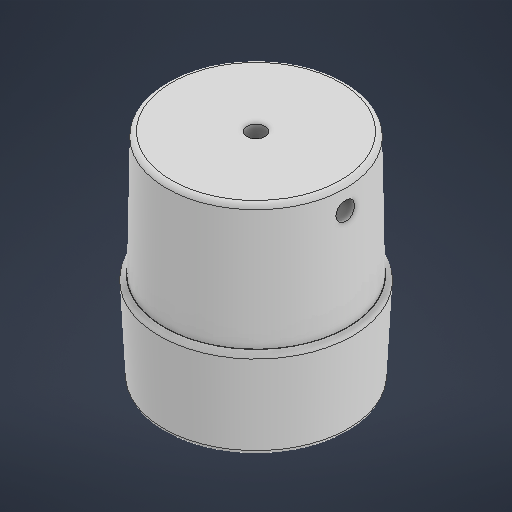
# Autodesk Inventor part: Part1
Saved by Autodesk Inventor 2025.2 (Build 292293000, 293)
## iProperties
Created: 2025-03-31
Part Number: Part1
Material: Generic
Document SubType Name: Modeling
Designer: mylap
Density: 1 g/cm^3
Appearance: Default
Author: mylap
## iProperties of the stored document Body_3DPrint.ipt
Created: 2025-03-31
Part Number: Body_3DPrint
Material: Generic
Document SubType Name: Modeling
Designer: mylap
Density: 1 g/cm^3
Appearance: Default
Author: mylap
Autodesk Inventor part; units mm, degrees
ref_plane "YZ Plane" through (0, 0, 0) normal (1, 0, 0) x (0, 1, 0)
ref_plane "XZ Plane" through (0, 0, 0) normal (0, 1, 0) x (-1, 0, 0)
sketch "Sketch1" plane through (0, 0, 0) normal (0, 0, 1) x (1, 0, 0)
  line L0 (3.6486, 85.3502) -> (47.5906, 85.3502) construction
  line L1 (47.5906, 85.3502) -> (47.5906, 3.7437) construction
  line L2 (47.5906, 3.7437) -> (3.6486, 3.7437) construction
  line L3 (3.6486, 3.7437) -> (3.6486, 85.3502) construction
  line L4 (38.1257, 32.1297) -> (38.7446, 44.3426)
  line L5 (38.0333, 44.3426) -> (37.7533, 60.8363)
  line L6 (25.8783, 44.547) -> (25.8783, 32.1297)
  line L7 (25.8783, 60.8363) -> (25.8783, 44.547)
  line L8 (38.1257, 32.1297) -> (25.8783, 32.1297)
  line L9 (37.7533, 60.8363) -> (25.8783, 60.8363)
  line L10 (38.7446, 44.3426) -> (25.8783, 44.3426)
  circle A0 centre (25.8783, 60.4553) radius 1.27
  point P0 (0, 0)
  point P1 (27.0898, 60.8363)
  point P2 (25.8783, 59.1853)
  dimension "d4" = 43.942
  dimension "d25" = 0.7112
  dimension "d37" = 2.54
  dimension "d43" = 0.381
  constraints: 14 end point, 3 horizontal, 3 point on line, 1 centre point, 1 perpendicular, 2 other
  measures "d4" distance between parallel lines of L1 L3
  measures "d25" distance from line of L4.end L5
  measures "d37" diameter of A0
  measures "d43" distance of L7.start A0.centre
revolve "Revolution2" add sketch "Sketch1" angle 360 about axis through (25.8783, 60.8363, 0) along (0, -1, 0) contours L8 L6 L10 L4 | L10 L6 L7 A0 L9 L5
fillet "Fillet1" radius 0.635 1 edges at (13.012, 44.3426, 0)
fillet "Fillet2" radius 0.635 1 edges at (13.631, 32.1297, 0)
fillet "Fillet3" radius 0.635 1 edges at (14.0033, 60.8363, 0)
ref_plane "Work Plane1" through (25.8783, 32.5107, 0) normal (0, -1, 0) x (1, 0, 0)
sketch "Sketch4" plane through (25.8783, 32.5107, 0) normal (0, -1, 0) x (1, 0, 0)
  line L0 (0, 0) -> (-12.2779, 0)
  circle A0 centre (0, 0) radius 12.2779 projected
  circle A1 centre (-6.139, 0) radius 1.27
  line L1 (0, 0) -> (12.2779, 0)
  circle A2 centre (6.139, 0) radius 1.27
  point P0 (-25.8783, 0)
  point P1 (-7.409, 0)
  point P2 (-4.869, 0)
  point P3 (7.409, 0)
  point P4 (4.869, 0)
  dimension "d49" = 2.54
  constraints: 4 end point, 2 centre point, 2 horizontal, 2 midpoint, 2 point on circle
  measures "d49" diameter of A1
revolve "Revolution4" cut sketch "Sketch4" angle 360 about axis through (25.8783, 32.5107, 0) along (-1, 0, 0) picked at (-5.8098, 0.382) picked at (5.7642, -0.1967) contours L0 A1 | L1 A2
sketch "Sketch6" plane through (0, 0, 0) normal (0, 0, 1) x (1, 0, 0)
  line L0 (37.7639, 60.2121) -> (38.0333, 44.3426) projected
  circle A0 centre (37.4265, 57.6449) radius 1.27
  line L1 (37.8075, 57.6449) -> (36.1565, 57.6449)
  line L2 (24.6668, 60.8363) -> (27.0898, 60.8363) projected
  line L3 (25.8783, 60.8363) -> (25.8783, 44.3426)
  line L4 (13.68, 44.3426) -> (38.0766, 44.3426) projected
  circle A1 centre (14.3302, 57.6449) radius 1.27
  line L5 (37.4265, 57.6449) -> (31.6244, 57.6449)
  line L6 (13.9927, 60.2121) -> (13.7233, 44.3426) projected
  line L7 (13.9233, 56.1237) -> (13.9834, 59.6649)
  line L8 (13.9491, 57.6449) -> (15.5999, 57.6169)
  point P0 (0, 0)
  point P1 (37.8109, 57.4453)
  point P2 (37.828, 56.4401)
  point P3 (13.9287, 56.4401)
  dimension "d55" = 2.54
  dimension "d56" = 0.381
  dimension "d57" = 0.381
  constraints: 10 end point, 5 point on line, 2 horizontal, 2 midpoint, 1 perpendicular, 1 symmetric about line, 1 vertical, 6 other
  measures "d56" distance from line of L0 L5.start
  measures "d57" distance from line of point (14.33, 57.645) L6
revolve "Revolution5" cut sketch "Sketch6" angle 360 about axis through (37.4265, 57.6449, 0) along (-1, 0, 0) picked at (15.036, 57.5284) picked at (37.6873, 57.2433) contours L6 L8 A1 | L0 A0 L1
body "Solid2"
